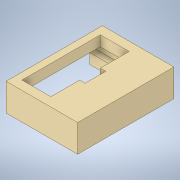
# Autodesk Inventor part: PCB_Holder_Compact
Saved by Autodesk Inventor 2020 (Build 240168000, 168)
## iProperties
Created: 2019-02-19
Part Number: PCB_Holder_Compact
Material: 일반
Document SubType Name: Modeling
Designer: Jeong Ji Hoon
Density: 1 g/cm^3
Appearance: 기본값
Author: Jeong Ji Hoon
## iProperties of the stored document _3D 인쇄.ipt
Created: 2019-08-13
Part Number: _3D 인쇄
Material: 일반
Document SubType Name: Modeling
Designer: Jeong Ji Hoon
Density: 1 g/cm^3
Appearance: 기본값
Author: Jeong Ji Hoon
Autodesk Inventor part; units mm, degrees
ref_plane "YZ Plane" through (0, 0, 0) normal (1, 0, 0) x (0, 1, 0)
ref_plane "XZ Plane" through (0, 0, 0) normal (0, 1, 0) x (-1, 0, 0)
ref_plane "XY Plane" through (0, 0, 0) normal (0, 0, 1) x (1, 0, 0)
sketch "스케치1" plane through (0, 0, 0) normal (0, 1, 0) x (-1, 0, 0)
  line L0 (0, 0) -> (0, -14)
  line L1 (0, -14) -> (10.4, -14)
  line L2 (0, 0) -> (10.4, 0)
  line L3 (10.4, 0) -> (10.4, -1.8)
  line L4 (10.4, -1.8) -> (5.2, -1.8)
  line L5 (5.2, -1.8) -> (5.2, -5.5)
  line L6 (5.2, -5.5) -> (4.4, -5.5)
  line L7 (4.4, -5.5) -> (4.4, -8.5)
  line L8 (4.4, -8.5) -> (5.2, -8.5)
  line L9 (5.2, -8.5) -> (5.2, -12.2)
  line L10 (5.2, -12.2) -> (10.4, -12.2)
  line L11 (10.4, -12.2) -> (10.4, -14)
  line L12 (10.4, -0.95) -> (4.4, -0.95) construction
  line L13 (4.4, -0.95) -> (4.4, -13.05) construction
  line L14 (4.4, -13.05) -> (10.4, -13.05) construction
  dimension "d0" = 14
  dimension "d2" = 10.4
  dimension "d3" = 1.8
  dimension "d5" = 3.7
  dimension "d6" = 0.8
  dimension "d7" = 3
  dimension "d8" = 0.8
  dimension "d9" = 3.7
  dimension "d47" = 12.1
  dimension "d48" = 0.85
  dimension "d49" = 0.85
  dimension "d63" = 6
  constraints: 30 end point, 5 horizontal, 5 vertical, 4 point on line, 3 perpendicular, 2 collinear
  measures "d0" distance of L0.start L0.end
  measures "d2" distance of L0.start L2.end
  measures "d3" distance of L2.end L3.end
  measures "d5" distance of L4.end L5.end
  measures "d6" distance of L5.end L6.end
  measures "d7" distance of L6.end L7.end
  measures "d8" distance of L7.end L8.end
  measures "d9" distance of L8.end L9.end
  measures "d47" distance between parallel lines of L14 L12
  measures "d48" distance between parallel lines of L12 L4
  measures "d49" distance between parallel lines of L10 L14
  measures "d63" distance between parallel lines of L13 L3
extrude "돌출1" add sketch "스케치1" along normal blind 4
sketch "스케치9" plane through (-10.4, 0, -14) normal (-1, 0, 0) x (0, 0, 1)
  line L0 (12.2, 0) -> (14, 0) projected
  line L1 (14, 0) -> (14, 4) projected
  line L2 (12.2, 4) -> (14, 4) projected
  line L3 (12.2, 0) -> (12.2, 4) projected
  line L4 (0, 0) -> (1.8, 0) projected
  line L5 (1.8, 0) -> (1.8, 4) projected
  line L6 (0, 4) -> (1.8, 4) projected
  line L7 (0, 0) -> (0, 4) projected
  line L8 (13.05, 1.5) -> (0.95, 1.5)
  line L9 (0.95, 1.5) -> (0.95, 2.5)
  line L10 (0.95, 2.5) -> (13.05, 2.5)
  line L11 (13.05, 2.5) -> (13.05, 1.5)
  dimension "d55" = 0.95
  dimension "d56" = 0.95
  dimension "d60" = 1
  dimension "d61" = 1.5
  dimension "d62" = 1.5
  dimension "d71" = 12.1
  constraints: 8 end point, 2 parallel, 1 horizontal, 1 perpendicular
  measures "d55" distance between parallel lines of L1 L11
  measures "d56" distance between parallel lines of L7 L9
  measures "d60" distance of L10.end L8.start
  measures "d61" distance between parallel lines of L0 L8
  measures "d62" distance between parallel lines of L2 L10
  measures "d71" distance of L9.end L10.end
extrude "돌출9" cut sketch "스케치9" against normal blind 6 contours L8 L5 L10 L3 | L3 L10 L11 L8 | L8 L9 L10 L5
sketch "스케치10" plane through (0, 4, 0) normal (0, 1, 0) x (1, 0, 0)
  line L0 (0, 0) -> (0, 14) projected
  line L1 (0, 14) -> (-10.4, 14) projected
  line L2 (-10.4, 14) -> (-10.4, 12.2) projected
  line L3 (-10.4, 12.2) -> (-5.2, 12.2) projected
  line L4 (-5.2, 12.2) -> (-5.2, 8.5) projected
  line L5 (-5.2, 8.5) -> (-4.4, 8.5) projected
  line L6 (-4.4, 8.5) -> (-4.4, 5.5) projected
  line L7 (-4.4, 5.5) -> (-5.2, 5.5) projected
  line L8 (-5.2, 5.5) -> (-5.2, 1.8) projected
  line L9 (-5.2, 1.8) -> (-10.4, 1.8) projected
  line L10 (-10.4, 1.8) -> (-10.4, 0) projected
  line L11 (-10.4, 0) -> (0, 0) projected
  line L12 (-5.2, 1.8) -> (-10.4, 1.8) projected
  line L13 (-5.2, 12.2) -> (-10.4, 12.2) projected
  line L14 (-10.4, 1.8) -> (-9.4, 1.8)
  line L15 (-9.4, 1.8) -> (-9.4, 12.2)
  line L16 (-9.4, 12.2) -> (-10.4, 12.2)
  line L17 (-10.4, 12.2) -> (-10.4, 1.8)
  point P0 (-9.4, 1.8)
  point P1 (-9.4, 12.2)
  dimension "d64" = 1
  constraints: 8 end point, 2 parallel, 1 horizontal, 1 perpendicular, 1 point on line
  measures "d64" distance of L16.end L15.end
extrude "돌출10" add sketch "스케치10" against normal up to surface (1.5 mm away) contours L17 L3 L15 L9
sketch "스케치11" plane through (0, 4, 0) normal (0, 1, 0) x (1, 0, 0)
  line L0 (-9.4, 1.3) -> (-5.2, 1.3)
  line L1 (-5.2, 1.3) -> (-5.2, 12.7)
  line L2 (-5.2, 12.7) -> (-9.4, 12.7)
  line L3 (-9.4, 12.7) -> (-9.4, 1.3)
  line L4 (-9.4, 1.8) -> (-9.4, 12.2) projected
  line L5 (-5.2, 12.2) -> (-5.2, 8.5) projected
  line L6 (-5.2, 1.8) -> (-9.4, 1.8) projected
  line L7 (-9.4, 12.2) -> (-5.2, 12.2) projected
  point P0 (0, 0)
  point P1 (-5.2, 12.2)
  dimension "d67" = 0.5
  dimension "d68" = 0.5
  constraints: 8 end point, 2 collinear, 2 parallel, 1 horizontal, 1 perpendicular
  measures "d67" distance between parallel lines of L0 L6
  measures "d68" distance between parallel lines of L7 L2
extrude "돌출11" cut sketch "스케치11" against normal up to surface (1.5 mm away) contours L3 L6 L1 L0 | L3 L2 L1 L7
equation "\"d5\" = d9"
equation "\"d9\" = 0.5 * d0 - 0.5 * d7 - d3"
equation "\"d48\" = d49"
equation "\"d55\" = d56"
equation "\"d61\" = d62"
